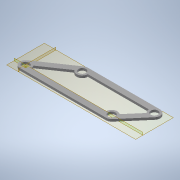
# Autodesk Inventor part: Plastic poging
Saved by Autodesk Inventor 2021 (Build 250183000, 183)
## iProperties
Manager: PJ / DCS
Company: Emmaüs Bovenbouw Aalter
Created: 2021-02-07
Part Number: Plastic poging
Material: S235
Catalog Web Link: http://emmausbovenbouw.op-weg.be/
Vendor: Emmaüsinstituut Bovenbouw Aalter
Document SubType Name: Modeling
Designer: Antho
Engineer: Declercq St.
Manufacturer: Standard
Standards Organization: Custom
Density: 7.86 g/cm^3
Appearance: Steel
Title: Algemene titel
Subject: Specifieke titel
Author: Antho
Keywords: Ruwe Ø xxxxx
Comments: Opmerking
Autodesk Inventor part; units mm, degrees
sketch "Sketch1" plane through (0, 0, 0) normal (0, 0, 1) x (1, 0, 0)
  line L0 (0, 39.622) -> (0, -39.622) construction
  line L1 (-80.0891, 0) -> (80.0891, 0) construction
  line L2 (0, 0) -> (191.205, 0)
  line L3 (191.205, 0) -> (235.078, 0)
  line L4 (235.078, 0) -> (235.078, 51)
  line L5 (191.205, 0) -> (235.078, 51)
  line L6 (0, 0) -> (74.795, 51)
  line L7 (74.795, 51) -> (235.078, 51)
  circle A0 centre (74.795, 51) radius 8
  circle A1 centre (235.078, 51) radius 8
  circle A2 centre (0, 0) radius 8
  circle A3 centre (0, 0) radius 12.5
  circle A4 centre (74.795, 51) radius 12.5
  circle A5 centre (235.078, 51) radius 12.5
  circle A6 centre (191.205, 0) radius 8
  circle A7 centre (191.205, 0) radius 12.5
  line L8 (0, -12.5) -> (191.205, -12.5)
  line L9 (67.4862, 61.1406) -> (-7.0415, 10.328)
  line L10 (245.078, 43.5) -> (200.6845, -8.148)
  line L11 (74.795, 63.5) -> (235.078, 63.5)
  point P0 (10.3276, 7.042)
  point P1 (64.4674, 43.958)
  point P2 (87.295, 51)
  point P3 (222.578, 51)
  point P4 (226.9261, 41.5239)
  point P5 (199.3569, 9.4761)
  point P6 (178.705, 0)
  point P7 (12.5, 0)
  dimension "d0" = 191.205
  dimension "d1" = 43.873
  dimension "d2" = 51
  dimension "d5" = 51
  dimension "d6" = 74.795
  dimension "d7" = 160.283
  dimension "d8" = 16
  dimension "d9" = 16
  dimension "d11" = 16
  dimension "d12" = 25
  dimension "d13" = 25
  dimension "d14" = 25
  dimension "d16" = 16
  dimension "d17" = 25
  constraints: 24 end point, 9 coincident, 8 centre point, 8 point on circle, 4 tangent, 3 horizontal, 2 midpoint, 2 vertical, 1 point on line
  measures "d0" distance of L2.start L2.end
  measures "d1" distance of L2.end L3.end
  measures "d2" distance of L3.end L4.end
  measures "d5" vertical distance of L2.start L6.end
  measures "d6" horizontal distance of L2.start L6.end
  measures "d7" distance of L6.end L4.end
  measures "d8" diameter of A0
  measures "d9" diameter of A1
  measures "d11" diameter of A2
  measures "d12" diameter of A3
  measures "d13" diameter of A4
  measures "d14" diameter of A5
  measures "d16" diameter of A6
  measures "d17" diameter of A7
extrude "Extrusion1" add sketch "Sketch1" along normal blind 5 contours A2 L6 A3 L2 | L2 A3 L6 A2 | L2 A7 L8 A3 | A3 L9 A4 L6 | A7 L5 A6 L2 | L2 A6 L3 A7 | A4 L7 A0 L6 | L6 A0 L7 A4 | A7 L3 A6 L5 | L5 A5 L4 L10 L3 A7 | A4 L11 A5 L7 | A5 L7 A1 L5 | L5 A1 L4 A5 | L3 L10 A7 | A5 L10 L4 A1 L7 | A5 L10 L4
body "Solid1"
